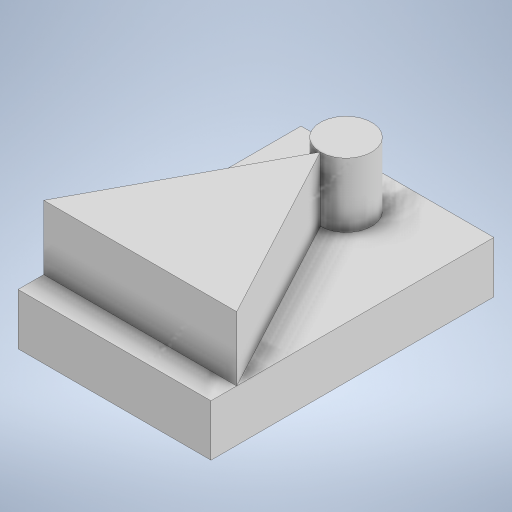
# Autodesk Inventor part: NOTGATE2
Saved by Autodesk Inventor 2024 (Build 280153000, 153)
## iProperties
Created: 2024-03-14
Part Number: NOTGATE2
Material: Generic
Document SubType Name: Modeling
Designer: Jonat
Density: 1 g/cm^3
Appearance: Default
Author: Jonat
Autodesk Inventor part; units mm, degrees
ref_plane "YZ Plane" through (0, 0, 0) normal (1, 0, 0) x (0, 1, 0)
ref_plane "XZ Plane" through (0, 0, 0) normal (0, 1, 0) x (-1, 0, 0)
ref_plane "XY Plane" through (0, 0, 0) normal (0, 0, 1) x (1, 0, 0)
sketch "Sketch1" plane through (0, 0, 0) normal (0, 1, 0) x (-1, 0, 0)
  line L0 (-6.5289, 0) -> (8.4711, 0)
  line L1 (0.9711, 32.1346) -> (0.9711, -29.0763) construction
  circle A0 centre (0.9711, -16) radius 2
  line L2 (8.4711, 0) -> (0.9711, -14)
  line L3 (-6.5289, 0) -> (0.9711, -14)
  point P0 (0, 0)
  point P1 (0.9711, -16.7566)
  dimension "d1" = 4
  dimension "d0" = 15
  dimension "d2" = 14
  constraints: 8 end point, 2 point on line, 1 coincident, 1 equal length, 1 horizontal, 1 vertical, 1 vertical alignment, 2 other
  measures "d0" distance of L0.start L0.end
  measures "d2" vertical distance of L0.end L2.end
extrude "Extrusion1" add sketch "Sketch1" along normal blind 5
sketch "Sketch2" plane through (0, 0, 0) normal (0, -1, 0) x (1, 0, 0)
  line L0 (-8.4711, 0) -> (6.5289, 0) projected
  line L1 (6.5289, 0) -> (-8.4711, 0)
  line L2 (-8.4711, 0) -> (-8.4711, -18)
  line L3 (-8.4711, -18) -> (6.5289, -18)
  line L4 (6.5289, -18) -> (6.5289, 0)
  line L5 (-8.4711, 0) -> (6.5289, 0)
  line L6 (6.5289, 0) -> (6.5289, 2)
  line L7 (6.5289, 2) -> (-8.4711, 2)
  line L8 (-8.4711, 2) -> (-8.4711, 0)
  line L9 (-8.4711, -18) -> (6.5289, -18)
  line L10 (6.5289, -18) -> (6.5289, -20)
  line L11 (6.5289, -20) -> (-8.4711, -20)
  line L12 (-8.4711, -20) -> (-8.4711, -18)
  point P0 (0, 0)
  dimension "d5" = 18
  dimension "d8" = 2
  constraints: 24 end point, 6 parallel, 3 horizontal, 3 perpendicular, 1 collinear
  measures "d5" distance of L2.end L1.end
  measures "d8" distance of L11.end L2.end
extrude "Extrusion2" add sketch "Sketch2" along normal blind 4
body "Solid1"
